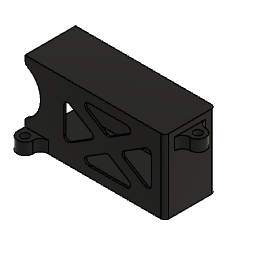
バッテリー固定具 (Autodesk Fusion 360 design; units mm, degrees)
Autodesk Fusion 360 part; units mm, degrees
note: some values were not read from the file. Set by a fixed rule: which sketch regions a step uses.
sketch "スケッチ1" plane through (0, 0, 0) normal (0, 0, 1) x (1, 0, 0)
  line L0 (0, 0) -> (36, 0)
  line L1 (36, 0) -> (36, 24)
  line L2 (36, 24) -> (0, 24)
  line L3 (0, 24) -> (0, 0)
  line L4 (-1, -1) -> (37, -1)
  line L5 (37, -1) -> (37, 25)
  line L6 (37, 25) -> (-1, 25)
  line L7 (-1, 25) -> (-1, -1)
  dimension "d1" = 36
  dimension "d2" = 24
  constraint horizontal L0
  constraint vertical L1
  constraint horizontal L2
  constraint vertical L3
  constraint coincident L0.start L3.end
  constraint horizontal L4
  constraint vertical L5
  constraint horizontal L6
  constraint vertical L7
  measures "d1" distance of L0.start L0.end
  measures "d2" distance of L0.start L2.end
extrude "押し出し1" add sketch "スケッチ1" along normal blind 72
sketch "スケッチ2" plane through (0, 0, 0) normal (0, 0, 1) x (1, 0, 0)
  line L0 (0, 24) -> (36, 24)
  line L1 (36, 24) -> (36, 0)
  line L2 (36, 0) -> (0, 0)
  line L3 (0, 0) -> (0, 24)
  constraint horizontal L0
  constraint vertical L1
  constraint horizontal L2
  constraint vertical L3
extrude "押し出し2" add sketch "スケッチ2" along normal blind 1
move_body "移動1" bodies 1 to x (0, 0, 1) y (0, 1, 0) z (-1, 0, 0) at (-1, 0, 1)
sketch "スケッチ3" plane through (0, 0, 0) normal (0, 0, -1) x (1, 0, 0)
  line L0 (-1, -25) -> (-1, 1)
  line L1 (-1, 1) -> (-73, 1)
  line L2 (-73, 1) -> (-73, -25)
  line L3 (-73, -25) -> (-1, -25)
  line L4 (-73, 1) -> (-65, 1)
  line L5 (-69, 1) -> (-69, 9)
  circle A0 centre (-69, 5) radius 2
  circle A1 centre (-69, 5) radius 4
  line L6 (-71, -29) -> (-70, -29)
  circle A2 centre (-69, -29) radius 4
  circle A3 centre (-69, -29) radius 2
  line L7 (-73, 5) -> (-73, 1)
  line L8 (-65, 5) -> (-65, 1)
  line L9 (-65, -25) -> (-65, -29)
  line L10 (-73, -25) -> (-73, -29)
  dimension "d7" = 8
  dimension "d8" = 8
  dimension "d9" = 4
  dimension "d10" = 8
  dimension "d11" = 4
  constraint coincident L1.end L2.start
  constraint perpendicular L2 L4
  constraint midpoint L4 L5.start
  constraint perpendicular L4 L5
  constraint midpoint L5 A0.centre
  constraint concentric A0 A1
  constraint perpendicular L2 L6
  constraint concentric A2 A3
  constraint coincident A1 L7.start
  constraint tangent A1 L7
  constraint coincident A1 L8.start
  constraint tangent A1 L8
  constraint coincident L3 L9.start
  constraint coincident A2 L9.end
  constraint tangent A2 L9
  constraint perpendicular L3 L9
  constraint coincident L2.end L3.start
  constraint coincident A2 L10.end
  constraint tangent A2 L10
  measures "d7" distance of L1.end L4.end
  measures "d8" distance of L5.start L5.end
  measures "d9" diameter of A0
  measures "d10" diameter of A1
  measures "d11" diameter of A3
extrude "押し出し3" add sketch "スケッチ3" against normal blind 6 contours L3 A2 L9 | L1 L4 A1 L8 | L3 A2 L10 | A2 | L5 A0 A1 | L1 L4 A1 L7 | L5 A0 A1
fillet "フィレット1" radius 4 2 edges at (-65, -1, 3) (-65, 25, 3)
sketch "スケッチ4" plane through (0, 0, 38) normal (0, 0, 1) x (-1, 0, 0)
  line L0 (1, 1) -> (1, -25)
  line L1 (1, -25) -> (73, -25)
  line L2 (73, -25) -> (73, 1)
  line L3 (73, 1) -> (1, 1)
  line L4 (1, -12) -> (-7, -12)
  circle A0 centre (-3, -12) radius 4
  circle A1 centre (-3, -12) radius 2
  line L5 (-3, -8) -> (1, -8)
  line L6 (-3, -16) -> (1, -16)
  constraint midpoint L0 L4.start
  constraint perpendicular L0 L4
  constraint midpoint L4 A0.centre
  constraint concentric A0 A1
  constraint coincident A0 L5.start
  constraint coincident L0 L5.end
  constraint tangent A0 L5
  constraint perpendicular L0 L5
  constraint coincident A0 L6.start
  constraint coincident L0 L6.end
  constraint tangent A0 L6
  constraint perpendicular L0 L6
extrude "押し出し4" add sketch "スケッチ4" against normal blind 6 contours L0 A0 L5 | L4 A0 A1 | L4 A0 A1 | L0 A0 L6
sketch "スケッチ5" plane through (0, 0, 38) normal (0, 0, 1) x (-1, 0, 0)
  circle A0 centre (-3, -12) radius 2
  line L0 (1, 1) -> (1, -8)
  line L1 (1, -8) -> (-3, -8)
  arc A1 (-3, -8) -> (-3, -16) centre (-3, -12) ccw
  line L2 (-3, -16) -> (1, -16)
  line L3 (1, -16) -> (1, -25)
  line L4 (1, -25) -> (73, -25)
  line L5 (73, -25) -> (73, 1)
  line L6 (73, 1) -> (1, 1)
  line L7 (1, -8) -> (1, -16)
  constraint coincident L0.end L1.start
  constraint coincident L2.end L3.start
extrude "押し出し5" cut sketch "スケッチ5" against normal blind 1.604 contours L1 A1 L2 L7
extrude "押し出し6" add 1 faces at (-0.3333, 12, 32) along direction (0, 0, -1) blind 1.604
fillet "フィレット2" radius 4 2 edges at (-1, 8, 33.396) (-1, 16, 33.396)
extrude "押し出し7" cut 1 faces at (-0.0924, 12, 36.396) along direction (0, 0, -1) blind 1.5
extrude "押し出し8" add 1 faces at (-0.0924, 12, 30.396) along direction (0, 0, -1) blind 1.5
fillet "フィレット3" radius 2 2 edges at (-1, 25, 19) (-1, -1, 19)
fillet "フィレット4" radius 2 2 edges at (-2, 24, 19) (-2, 0, 19)
sketch "スケッチ6" plane through (0, -1, 0) normal (0, -1, 0) x (1, 0, 0)
  line L0 (-3, 0) -> (-3, 38)
  line L1 (-3, 38) -> (-73, 38)
  line L2 (-73, 38) -> (-73, 6)
  line L3 (-73, 6) -> (-61, 6)
  line L4 (-61, 6) -> (-61, 0)
  line L5 (-61, 0) -> (-3, 0)
  line L6 (-73, 22) -> (-53, 22)
  line L7 (-3, 22) -> (-13, 22)
  line L8 (-13, 38) -> (-13, 30)
  line L9 (-13, 0) -> (-13, 8)
  line L10 (-53, 22) -> (-53, 23)
  line L11 (-53, 23) -> (-53, 30)
  line L12 (-53, 30) -> (-13, 30)
  line L13 (-13, 8) -> (-13, 30)
  line L14 (-13, 8) -> (-53, 8)
  line L15 (-53, 8) -> (-53, 22)
  line L16 (-53, 8) -> (-13, 30)
  line L17 (-33, 19) -> (-31.7952, 16.8095)
  line L18 (-33, 19) -> (-34.2048, 21.1905)
  line L19 (-34.2048, 21.1905) -> (-18.1876, 30)
  line L20 (-31.7952, 16.8095) -> (-13, 27.1468)
  line L21 (-31.7952, 16.8095) -> (-47.8124, 8)
  line L22 (-34.2048, 21.1905) -> (-53, 10.8532)
  line L23 (-13, 30) -> (-13, 33)
  line L24 (-13, 33) -> (-8, 33)
  line L25 (-8, 33) -> (-8, 3)
  line L26 (-13, 8) -> (-13, 5)
  line L27 (-8, 5) -> (-13, 5)
  line L28 (-53, 30) -> (-53, 33)
  line L29 (-53, 33) -> (-13, 33)
  line L30 (-53, 8) -> (-53, 5)
  line L31 (-53, 5) -> (-13, 5)
  dimension "d32" = 2.5
  dimension "d33" = 2.5
  dimension "d34" = 3
  dimension "d35" = 5
  constraint midpoint L2 L6.start
  constraint perpendicular L2 L6
  constraint coincident L0 L7.start
  constraint perpendicular L0 L7
  constraint coincident L1 L8.start
  constraint perpendicular L1 L8
  constraint coincident L5 L9.start
  constraint perpendicular L5 L9
  constraint perpendicular L6 L10
  constraint perpendicular L6 L11
  constraint perpendicular L8 L12
  constraint perpendicular L12 L13
  constraint perpendicular L13 L14
  constraint perpendicular L6 L15
  constraint midpoint L16 L17.start
  constraint perpendicular L16 L17
  constraint perpendicular L16 L18
  constraint coincident L12 L19.end
  constraint perpendicular L18 L19
  constraint coincident L13 L20.end
  constraint perpendicular L17 L20
  constraint coincident L14 L21.end
  constraint perpendicular L17 L21
  constraint coincident L15 L22.end
  constraint perpendicular L18 L22
  constraint coincident L8 L23.end
  constraint perpendicular L23 L24
  constraint perpendicular L7 L25
  constraint coincident L9 L26.end
  constraint perpendicular L14 L26
  constraint coincident L25 L27.start
  constraint perpendicular L9 L27
  constraint perpendicular L12 L28
  constraint perpendicular L8 L29
  constraint perpendicular L14 L30
  constraint perpendicular L26 L31
  measures "d32" distance of L17.start L17.end
  measures "d33" distance of L17.start L18.end
  measures "d34" distance of L8.end L23.end
  measures "d35" distance of L23.end L24.end
extrude "押し出し9" cut sketch "スケッチ6" against normal blind 98 contours L7 L9 L13 L25 L26 L27 | L7 L8 L13 L23 L24 L25 | L9 L14 L26 L30 L31 | L13 L14 L20 L21 | L8 L12 L23 L28 L29 | L13 L16 L17 L20 | L14 L16 L17 L21 | L15 L16 L18 L22 | L12 L16 L18 L19 | L10 L11 L12 L15 L19 L22
sketch "スケッチ7" plane through (0, -1, 0) normal (0, -1, 0) x (1, 0, 0)
  line L0 (-8, 5) -> (-53, 5)
  line L1 (-53, 5) -> (-53, 33)
  line L2 (-53, 33) -> (-8, 33)
  line L3 (-8, 33) -> (-8, 5)
  line L4 (-3, 0) -> (-3, 38)
  line L5 (-3, 38) -> (-73, 38)
  line L6 (-73, 38) -> (-73, 6)
  line L7 (-73, 6) -> (-61, 6)
  line L8 (-61, 6) -> (-61, 0)
  line L9 (-61, 0) -> (-3, 0)
  line L10 (-53, 33) -> (-8, 5)
  line L11 (-30.5, 19) -> (-28.9151, 21.5472)
  line L12 (-30.5, 19) -> (-32.0849, 16.4528)
  line L13 (-32.0849, 16.4528) -> (-53, 29.4667)
  line L14 (-28.9151, 21.5472) -> (-47.3214, 33)
  line L15 (-28.9151, 21.5472) -> (-8, 8.5333)
  line L16 (-32.0849, 16.4528) -> (-13.6786, 5)
  dimension "d38" = 3
  dimension "d39" = 3
  constraint coincident L1.end L2.start
  constraint coincident L0.start L3.end
  constraint midpoint L10 L11.start
  constraint perpendicular L10 L11
  constraint perpendicular L10 L12
  constraint coincident L1 L13.end
  constraint perpendicular L12 L13
  constraint coincident L2 L14.end
  constraint perpendicular L11 L14
  constraint coincident L3 L15.end
  constraint perpendicular L11 L15
  constraint coincident L0 L16.end
  constraint perpendicular L12 L16
  measures "d38" distance of L11.start L11.end
  measures "d39" distance of L11.start L12.end
extrude "押し出し10" add sketch "スケッチ7" against normal blind 26 contours L3 L10 L11 L15 | L0 L10 L12 L16 | L1 L10 L12 L13 | L2 L10 L11 L14
sketch "スケッチ8" plane through (-73, 0, 0) normal (-1, 0, 0) x (0, -1, 0)
  line L0 (0, 1) -> (-24, 1)
  line L1 (-24, 1) -> (-24, 37)
  line L2 (-24, 37) -> (0, 37)
  line L3 (0, 37) -> (0, 1)
  line L4 (-25, 0) -> (5, 0)
  line L5 (5, 0) -> (5, 6)
  line L6 (5, 6) -> (1, 6)
  line L7 (1, 6) -> (1, 38)
  line L8 (1, 38) -> (-25, 38)
  line L9 (-25, 38) -> (-25, 6)
  line L10 (-25, 6) -> (-25, 0)
extrude "押し出し11" cut sketch "スケッチ8" against normal blind 66 contours L0 L1 L2 L3
sketch "スケッチ9" plane through (0, -1, 0) normal (0, -1, 0) x (1, 0, 0)
  line L0 (-13.6786, 5) -> (-53, 5)
  line L1 (-53, 5) -> (-53, 29.4667)
  line L2 (-53, 29.4667) -> (-13.6786, 5)
  line L3 (-8, 8.5333) -> (-47.3214, 33)
  line L4 (-47.3214, 33) -> (-8, 33)
  line L5 (-8, 33) -> (-8, 8.5333)
  line L6 (-3, 0) -> (-3, 38)
  line L7 (-3, 38) -> (-73, 38)
  line L8 (-73, 38) -> (-73, 6)
  line L9 (-73, 6) -> (-61, 6)
  line L10 (-61, 6) -> (-61, 0)
  line L11 (-61, 0) -> (-3, 0)
  line L12 (-53, 5) -> (-8, 33)
  line L13 (-30.5, 19) -> (-28.9151, 16.4528)
  line L14 (-28.9151, 16.4528) -> (-32.0849, 21.5472)
  line L15 (-32.0849, 21.5472) -> (-13.6786, 33)
  line L16 (-28.9151, 16.4528) -> (-8, 29.4667)
  line L17 (-28.9151, 16.4528) -> (-47.3214, 5)
  line L18 (-32.0849, 21.5472) -> (-53, 8.5333)
  dimension "d44" = 3
  dimension "d45" = 6
  constraint coincident L0.end L1.start
  constraint coincident L4.end L5.start
  constraint midpoint L12 L13.start
  constraint perpendicular L12 L13
  constraint perpendicular L12 L14
  constraint coincident L4 L15.end
  constraint perpendicular L13 L15
  constraint coincident L5 L16.end
  constraint perpendicular L13 L16
  constraint coincident L0 L17.end
  constraint perpendicular L14 L17
  constraint coincident L1 L18.end
  constraint perpendicular L14 L18
  measures "d44" distance of L13.start L13.end
  measures "d45" distance of L13.end L14.end
extrude "押し出し12" add sketch "スケッチ9" against normal blind 26 contours L0 L2 L12 L17 | L1 L2 L12 L18 | L3 L5 L12 L16 | L3 L4 L12 L15
sketch "スケッチ10" plane through (-73, 0, 0) normal (-1, 0, 0) x (0, -1, 0)
  line L0 (0, 1) -> (-24, 1)
  line L1 (-24, 1) -> (-24, 37)
  line L2 (-24, 37) -> (0, 37)
  line L3 (0, 37) -> (0, 1)
  line L4 (-25, 0) -> (5, 0)
  line L5 (5, 0) -> (5, 6)
  line L6 (5, 6) -> (1, 6)
  line L7 (1, 6) -> (1, 38)
  line L8 (1, 38) -> (-25, 38)
  line L9 (-25, 38) -> (-25, 6)
  line L10 (-25, 6) -> (-25, 0)
extrude "押し出し13" cut sketch "スケッチ10" against normal blind 66 contours L0 L1 L2 L3
fillet "フィレット5" radius 2 3 edges at (-13.6786, -0.5, 33) (-47.3214, -0.5, 33) (-30.5, -0.5, 22.5333)
fillet "フィレット6" radius 2 9 edges at (-24.8214, -0.5, 19) (-47.3214, -0.5, 5) (-13.6786, -0.5, 5) (-8, -0.5, 8.5333) (-8, -0.5, 29.4667) (-30.5, -0.5, 15.4667) (-36.1786, -0.5, 19) (-53, -0.5, 8.5333) (-53, -0.5, 29.4667)
fillet "フィレット7" radius 2 12 edges at (-30.5, 24.5, 22.5333) (-24.8214, 24.5, 19) (-47.3214, 24.5, 33) (-36.1786, 24.5, 19) (-13.6786, 24.5, 33) (-53, 24.5, 29.4667) (-53, 24.5, 8.5333) (-8, 24.5, 29.4667) (-8, 24.5, 8.5333) (-30.5, 24.5, 15.4667) (-47.3214, 24.5, 5) (-13.6786, 24.5, 5)
sketch "スケッチ11" plane through (0, -1, 0) normal (0, -1, 0) x (1, 0, 0)
  line L0 (-8, 25.8667) -> (-8, 12.1333)
  arc A0 (-11.0566, 10.4352) -> (-8, 12.1333) centre (-10, 12.1333) ccw
  line L1 (-11.0566, 10.4352) -> (-22.0923, 17.3019)
  arc A1 (-22.0923, 20.6981) -> (-22.0923, 17.3019) centre (-21.0357, 19) ccw
  line L2 (-22.0923, 20.6981) -> (-11.0566, 27.5648)
  arc A2 (-8, 25.8667) -> (-11.0566, 27.5648) centre (-10, 25.8667) ccw
  line L3 (-53, 12.1333) -> (-53, 25.8667)
  arc A3 (-49.9434, 27.5648) -> (-53, 25.8667) centre (-51, 25.8667) ccw
  line L4 (-49.9434, 27.5648) -> (-38.9077, 20.6981)
  arc A4 (-38.9077, 17.3019) -> (-38.9077, 20.6981) centre (-39.9643, 19) ccw
  line L5 (-38.9077, 17.3019) -> (-49.9434, 10.4352)
  arc A5 (-53, 12.1333) -> (-49.9434, 10.4352) centre (-51, 12.1333) ccw
  arc A6 (-29.4434, 14.8092) -> (-31.5566, 14.8092) centre (-30.5, 13.1111) ccw
  line L6 (-29.4434, 14.8092) -> (-19.622, 8.6981)
  arc A7 (-20.6786, 5) -> (-19.622, 8.6981) centre (-20.6786, 7) ccw
  line L7 (-20.6786, 5) -> (-40.3214, 5)
  arc A8 (-41.378, 8.6981) -> (-40.3214, 5) centre (-40.3214, 7) ccw
  line L8 (-41.378, 8.6981) -> (-31.5566, 14.8092)
  arc A9 (-31.5566, 23.1908) -> (-29.4434, 23.1908) centre (-30.5, 24.8889) ccw
  line L9 (-31.5566, 23.1908) -> (-41.378, 29.3019)
  arc A10 (-40.3214, 33) -> (-41.378, 29.3019) centre (-40.3214, 31) ccw
  line L10 (-40.3214, 33) -> (-20.6786, 33)
  arc A11 (-19.622, 29.3019) -> (-20.6786, 33) centre (-20.6786, 31) ccw
  line L11 (-19.622, 29.3019) -> (-29.4434, 23.1908)
  line L12 (-3, 0) -> (-3, 38)
  line L13 (-3, 38) -> (-73, 38)
  line L14 (-73, 38) -> (-73, 6)
  line L15 (-73, 6) -> (-61, 6)
  line L16 (-61, 6) -> (-61, 0)
  line L17 (-61, 0) -> (-3, 0)
  line L18 (-73, 38) -> (-73, 34)
  line L19 (-73, 6) -> (-73, 10)
  line L20 (-73, 34) -> (-73, 10)
  line L21 (-73, 22) -> (-63, 22)
  circle A12 centre (-78, 22) radius 13
  constraint coincident L13.end L14.start
  constraint coincident L14 L18.end
  constraint perpendicular L13 L18
  constraint coincident L14.end L15.start
  constraint coincident L14 L19.end
  constraint perpendicular L15 L19
  constraint parallel L14 L20
  constraint midpoint L14 L21.start
  constraint perpendicular L14 L21
  constraint coincident L18.end A12
extrude "押し出し14" cut sketch "スケッチ11" against normal blind 40 contours L14 L20 L21 A12 | L14 L20 L21 A12
fillet "フィレット8" radius 2 4 edges at (-73, 24.5, 34) (-73, -0.5, 34) (-73, -0.5, 10) (-73, 24.5, 10)
